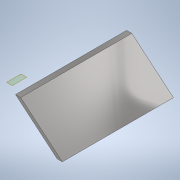
# Autodesk Inventor part: mirror
Saved by Autodesk Inventor 2022 (Build 260153000, 153)
## iProperties
Created: 2022-12-26
Part Number: mirror
Material: Steel, Alloy
Document SubType Name: Modeling
Designer: Kamil
Density: 7.73 g/cm^3
Appearance: Semi-Polished
Author: Kamil
Autodesk Inventor part; units mm, degrees
ref_plane "YZ Plane" through (0, 0, 0) normal (1, 0, 0) x (0, 1, 0)
ref_plane "XZ Plane" through (0, 0, 0) normal (0, 1, 0) x (-1, 0, 0)
ref_plane "XY Plane" through (0, 0, 0) normal (0, 0, 1) x (1, 0, 0)
sketch "Sketch1" plane through (0, 0, 0) normal (0, 0, 1) x (1, 0, 0)
  line L0 (-44.6274, 16.55) -> (3.1619, -23.55) projected
  line L1 (44.6274, -23.55) -> (3.1619, -23.55) projected
  line L2 (44.6274, -23.55) -> (44.6274, -12.55) projected
  line L3 (44.6274, -12.55) -> (28.5274, -12.55) projected
  arc A0 (10.4274, 5.55) -> (28.5274, -12.55) centre (28.5274, 5.55) ccw projected
  line L4 (10.4274, 5.55) -> (10.4274, 16.55) projected
  line L5 (10.4274, 16.55) -> (-44.6274, 16.55) projected
  line L6 (-55.3726, 21.65) -> (-32.3912, 2.3664) projected
  line L7 (-32.3912, 2.3664) -> (-30.4629, 4.6645) projected
  line L8 (-30.4629, 4.6645) -> (-50.7054, 21.65) projected
  line L9 (-50.7054, 21.65) -> (-55.3726, 21.65) projected
  line L10 (-32.3912, 2.3664) -> (12.526, -35.3237)
  line L11 (3.1619, -23.55) -> (14.4544, -33.0256)
  line L12 (14.4544, -33.0256) -> (12.526, -35.3237)
  point P0 (0, 0)
  constraints: 6 end point, 1 perpendicular
ref_plane "Work Plane1" through (-44.6274, -23.55, -100) normal (0, 0, -1) x (0, 1, 0)
extrude "Extrusion1" add sketch "Sketch1" against normal up to surface (100 mm away) contours L0 L11 L12 L10 L7
sketch "Sketch2" plane through (14.4544, -33.0256, -100) normal (0, 0, -1) x (-0.7660444, 0.6427876, 0)
  line L0 (-13.6181, 16.6167) -> (-12.086, 15.3311)
  line L1 (-12.086, 15.3311) -> (12.4819, -5.2838)
  line L2 (0, 0) -> (58.6353, 0) projected
  line L3 (0, -3) -> (0, 0) projected
  line L4 (58.6353, -3) -> (0, -3) projected
  line L5 (58.6353, 0) -> (58.6353, -3) projected
  point P0 (32.3011, 16.0079)
  point P1 (9.7601, -3)
  point P2 (6.1849, 0)
  constraints: 4 end point, 3 other
extrude "Extrusion2" cut sketch "Sketch2" against normal through all contours L1 L4 L3 L2
ref_plane "Work Plane2" through (-55.2717, 8.4367, -43.1782) normal (0, -1, 0) x (1, 0, 0)
sketch "Sketch4" plane through (-32.3912, 2.3664, -100) normal (-0.6427876, -0.7660444, 0) x (0.7660444, -0.6427876, 0)
  line L0 (48.8752, 0) -> (48.8752, 100) projected
  line L1 (0, 100) -> (48.8752, 100) projected
  line L2 (0, 100) -> (0, 0) projected
  line L3 (0, 0) -> (48.8752, 0) projected
  line L4 (-5.8685, 94) -> (-21.784, 94)
  line L5 (43.894, 94) -> (0.9766, 94)
  line L6 (48.8752, 0) -> (48.8752, 100) projected
  line L7 (48.8752, 50) -> (0, 50)
  line L8 (0, 100) -> (0, 0) projected
  line L9 (26.3342, 100) -> (26.3342, 94)
  line L10 (26.3342, 97) -> (26.3342, 96.5)
  circle A0 centre (26.3342, 96.5) radius 1.5
  circle A1 centre (26.3342, 3.5) radius 1.5
  dimension "d6" = 0.5
  dimension "d7" = 3
  constraints: 10 end point, 3 midpoint, 2 centre point, 2 horizontal, 2 point on line, 1 coincident, 1 perpendicular, 1 symmetric about line, 5 other
  measures "d6" distance of L10.start L10.end
  measures "d7" diameter of A0
extrude "Extrusion3" cut sketch "Sketch4" against normal blind 10 contours L9 A0 | L9 A0 | A1
chamfer "Chamfer1" distance 1 angle 45 2 edges at (-13.3671, -13.5967, -3.5) (-13.3671, -13.5967, -96.5)
body "Solid1"
